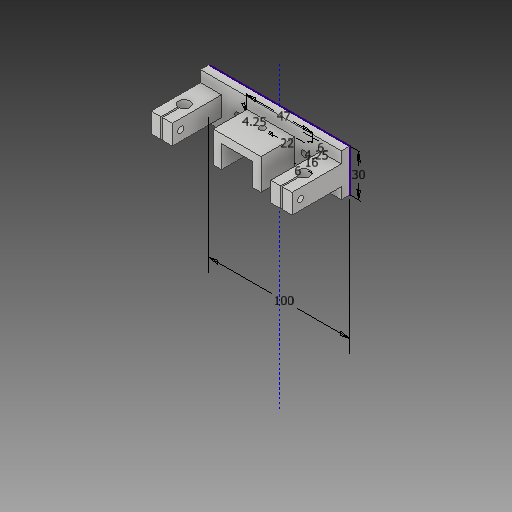
# Autodesk Inventor part: YPulleySupportBase
Saved by Autodesk Inventor 2019 (Build 230136000, 136)
## iProperties
Created: 2019-08-21
Part Number: YPulleySupportBase
Material: Generic
Document SubType Name: Modeling
Designer: Bruno
Density: 1 g/cm^3
Appearance: Default
Author: Bruno
Autodesk Inventor part; units mm, degrees
ref_plane "YZ Plane" through (0, 0, 0) normal (1, 0, 0) x (0, 1, 0)
ref_plane "XZ Plane" through (0, 0, 0) normal (0, 1, 0) x (-1, 0, 0)
ref_plane "XY Plane" through (0, 0, 0) normal (0, 0, 1) x (1, 0, 0)
sketch "Sketch1" plane through (0, 0, 0) normal (0, 0, 1) x (1, 0, 0)
  line L0 (50, 188.2731) -> (-50, 188.2731)
  line L1 (-50, 188.2731) -> (-50, 158.2731)
  line L2 (50, 158.2731) -> (50, 188.2731)
  line L3 (11, 158.2731) -> (11, 174.2731)
  line L4 (11, 174.2731) -> (-11, 174.2731)
  line L5 (-11, 174.2731) -> (-11, 158.2731)
  line L6 (17, 158.2731) -> (17, 180.2731)
  line L7 (17, 180.2731) -> (-17, 180.2731)
  line L8 (-17, 180.2731) -> (-17, 158.2731)
  line L9 (17, 158.2731) -> (50, 158.2731)
  line L10 (11, 158.2731) -> (17, 158.2731)
  line L11 (-11, 158.2731) -> (-17, 158.2731)
  line L12 (-17, 158.2731) -> (-50, 158.2731)
  circle A0 centre (23.5, 173.2731) radius 2.125
  circle A1 centre (-23.5, 173.2731) radius 2.125
  line L13 (0, 0) -> (0, 215.8038) construction
  line L14 (0, 158.2731) -> (11, 158.2731) construction
  line L15 (0, 158.2731) -> (-11, 158.2731) construction
  line L16 (-23.5, 173.2731) -> (23.5, 173.2731) construction
  line L17 (-23.5, 173.2731) -> (-23.5, 188.2731) construction
  line L18 (-23.5, 173.2731) -> (-23.5, 158.2731) construction
  dimension "d1" = 30
  dimension "d2" = 100
  dimension "d3" = 22
  dimension "d4" = 6
  dimension "d5" = 16
  dimension "d6" = 6
  dimension "d11" = 4.25
  dimension "d13" = 4.25
  dimension "d18" = 47
  constraints: 38 end point, 8 horizontal, 7 perpendicular, 5 equal length, 3 point on line, 3 vertical, 2 centre point, 1 collinear, 1 parallel, 1 symmetric about line
  measures "d1" distance of L2.start L0.start
  measures "d2" distance of L1.end L2.start
  measures "d3" distance of L3.end L4.end
  measures "d4" distance of L3.start L6.start
  measures "d5" distance of L3.start L3.end
  measures "d6" distance between parallel lines of L7 L4
  measures "d11" diameter of A0
  measures "d13" diameter of A1
  measures "d18" distance of L16.start L16.end
extrude "Extrusion1" add sketch "Sketch1" along normal blind 6 contours L2 L9 L6 L7 L8 L12 L1 L0
extrude "Extrusion2" add sketch "Sketch1" along normal blind 30 contours L10 L3 L4 L5 L11 L8 L7 L6
sketch "Sketch2" plane through (-17, 180.2731, 6) normal (0, 1, 0) x (1, 0, 0)
  circle A0 centre (16.8713, -6) radius 2.125
  line L0 (16.8713, -6) -> (33.9314, -6) construction
  line L1 (16.8713, -6) -> (-0.1889, -6) construction
  line L2 (67, 6) -> (-33, 6) projected
  point P0 (17, 6)
  dimension "d14" = 4.25
  dimension "d15" = 12
  constraints: 4 end point, 2 horizontal, 1 centre point, 1 collinear
  measures "d14" diameter of A0
  measures "d15" distance from line of L2 L0.start
extrude "Extrusion3" cut sketch "Sketch2" against normal up to next
sketch "Sketch3" plane through (0, 0, 6) normal (0, 0, 1) x (1, 0, 0)
  line L0 (50, 158.2731) -> (50, 188.2731) projected
  line L1 (50, 180.2731) -> (35, 180.2731)
  line L2 (35, 180.2731) -> (35, 166.2731)
  line L3 (35, 166.2731) -> (50, 166.2731)
  line L4 (43.2299, 188.2731) -> (43.2299, 180.2731) construction
  line L5 (43.4666, 166.2731) -> (43.4666, 158.2731) construction
  line L6 (50, 188.2731) -> (-50, 188.2731) projected
  line L7 (17, 158.2731) -> (50, 158.2731) projected
  line L8 (-50, 188.2731) -> (-50, 158.2731) projected
  line L9 (-50, 180.2731) -> (-35, 180.2731)
  line L10 (-35, 180.2731) -> (-35, 166.2731)
  line L11 (-35, 166.2731) -> (-50, 166.2731)
  line L12 (-50, 166.2731) -> (-50, 180.2731)
  point P0 (0, 0)
  dimension "d19" = 15
  dimension "d20" = 14
  constraints: 18 end point, 7 point on line, 4 perpendicular, 2 collinear, 2 equal length, 2 horizontal, 2 parallel, 1 vertical
  measures "d19" distance between parallel lines of L0 L2
  measures "d20" distance between parallel lines of L3 L1
extrude "Extrusion4" add sketch "Sketch3" along normal blind 35
sketch "Sketch4" plane through (35, 180.2731, 6) normal (0, 1, 0) x (1, 0, 0)
  circle A0 centre (7.5, -19) radius 4
  line L0 (7.5, -19) -> (15, -19) construction
  line L1 (15, 0) -> (15, -35) projected
  line L2 (7.5, -19) -> (0, -19) construction
  line L3 (0, 0) -> (0, -35) projected
  line L4 (15, 6) -> (-85, 6) projected
  line L5 (8, -22.9686) -> (8, -35)
  line L6 (7, -22.9686) -> (7, -35)
  line L7 (8, -37.8452) -> (15, -37.8452) construction
  line L8 (7, -37.8452) -> (0, -37.8452) construction
  circle A1 centre (-77.5, -19) radius 4
  line L9 (-85, -35) -> (-70, -35) projected
  line L10 (-78, -22.9686) -> (-78, -35)
  line L11 (-77, -37.6694) -> (-70, -37.6694) construction
  line L12 (-78, -37.628) -> (-85, -37.628) construction
  line L13 (-85, 0) -> (-85, -35) projected
  line L14 (-70, 0) -> (-70, -35) projected
  line L15 (-77, -22.9686) -> (-77, -35)
  line L16 (-77.5, -19) -> (-70, -19) construction
  line L17 (-77.5, -19) -> (-85, -19) construction
  line L18 (-77, -35) -> (-78, -35)
  line L19 (8, -35) -> (7, -35)
  line L20 (0, -35) -> (15, -35) projected
  point P0 (-35, 6)
  dimension "d23" = 8
  dimension "d24" = 25
  dimension "d25" = 1
  dimension "d26" = 8
  dimension "d27" = 1
  constraints: 28 end point, 17 point on line, 4 collinear, 4 equal length, 4 horizontal, 4 point on circle, 4 vertical, 2 centre point, 2 perpendicular
  measures "d23" diameter of A0
  measures "d24" distance between parallel lines of L4 L2
  measures "d25" distance between parallel lines of L5 L6
  measures "d26" diameter of A1
  measures "d27" distance between parallel lines of L10 L15
extrude "Extrusion5" cut sketch "Sketch4" against normal up to next
sketch "Sketch5" plane through (-50, 158.2731, 0) normal (-1, 0, 0) x (0, 0, 1)
  circle A0 centre (34.9843, 15) radius 2.125
  line L0 (0, 30) -> (0, 0) projected
  line L1 (34.9843, 15) -> (34.9843, 22)
  line L2 (6, 22) -> (41, 22) projected
  line L3 (34.9843, 15) -> (34.9843, 8)
  line L4 (6, 8) -> (41, 8) projected
  line L5 (34.9843, 15) -> (28.9686, 15)
  line L6 (34.9843, 15) -> (41, 15)
  line L7 (41, 22) -> (41, 8) projected
  line L8 (28.9686, 22) -> (28.9686, 8) projected
  point P0 (0, -158.2731)
  dimension "d30" = 4.25
  constraints: 8 end point, 2 collinear, 2 horizontal, 2 midpoint, 2 point on line, 2 vertical, 1 centre point
  measures "d30" diameter of A0
extrude "Extrusion6" cut sketch "Sketch5" against normal through all contours L6 L1 A0 | A0 L3 L6 | L1 L5 A0 | A0 L5 L3
body "Solid1"
